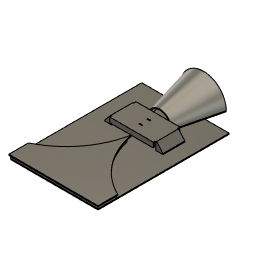
Constructed Color Sorter v1 (Autodesk Fusion 360 design; units mm, degrees)
Autodesk Fusion 360 part; units mm, degrees
sketch "Sketch1" plane through (0, 0, 0) normal (0, 1, 0) x (1, 0, 0)
  line L0 (0, 0) -> (304.8, 0)
  line L1 (304.8, 0) -> (304.8, 457.2)
  line L2 (304.8, 457.2) -> (0, 457.2)
  line L3 (0, 457.2) -> (0, 0)
  dimension "d1" = 304.8
  dimension "d2" = 457.2
  constraint horizontal L0
  constraint vertical L1
  constraint horizontal L2
  constraint vertical L3
  constraint coincident L0.start L3.end
  measures "d1" distance of L0.start L0.end
  measures "d2" distance of L0.start L2.end
extrude "Extrude1" add sketch "Sketch1" along normal blind 3.175 makes body 1
sketch "Sketch1 (2)" plane through (0, 0, 0) normal (0, 0, 1) x (1, 0, 0) in component "Ramp for Checkers v1"
  line L0 (0, 0) -> (0, 254) construction
  line L1 (0, 0) -> (152.4, 0)
  line L2 (152.4, 0) -> (152.4, 63.5)
  arc A0 (0, 254) -> (152.4, 63.5) centre (278.7714, 320.8071) ccw
  arc A1 (-152.4, 63.5) -> (0, 254) centre (-278.7714, 320.8071) ccw
  line L3 (-152.4, 0) -> (-152.4, 63.5)
  line L4 (0, 0) -> (-152.4, 0)
  dimension "d1_1" = 254
  dimension "d2_1" = 152.4
  dimension "d3_1" = 63.5
  constraint coincident L0.start L1.start
  constraint vertical L0
  constraint perpendicular L0 L1
  constraint perpendicular L1 L2
  constraint symmetric A0.start L0 A1.end
  constraint symmetric L0 L1.start L4.start
  constraint symmetric L0 L1.end L3.start
  constraint symmetric L0 L2.end A1.start
  constraint symmetric L0 A0 A1
  measures "d1_1" distance of L0.start L0.end
  measures "d2_1" distance of L0.start L1.end
  measures "d3_1" distance of L1.end L2.end
extrude "Extrude1'" add sketch "Sketch1 (2)" along normal blind 9.525 separate body makes body 2 in component "Ramp for Checkers v1"
sketch "Sketch2" plane through (0, 0, 9.525) normal (0, 0, 1) x (1, 0, 0) in component "Ramp for Checkers v1"
  line L0 (152.4, 0) -> (152.4, 63.5)
  arc A0 (0, 254) -> (152.4, 63.5) centre (278.7714, 320.8071) ccw
  arc A1 (-152.4, 63.5) -> (0, 254) centre (-278.7714, 320.8071) ccw
  line L1 (-152.4, 63.5) -> (-152.4, 0)
  line L2 (-152.4, 0) -> (152.4, 0)
  line L3 (155.575, -3.175) -> (155.575, 65.4856)
  arc A2 (0, 269.3003) -> (155.575, 65.4856) centre (278.7714, 320.8071) ccw
  arc A3 (-155.575, 65.4856) -> (0, 269.3003) centre (-278.7714, 320.8071) ccw
  line L4 (-155.575, 65.4856) -> (-155.575, -3.175)
  line L5 (-155.575, -3.175) -> (155.575, -3.175)
  dimension "d6" = -3.175
extrude "Extrude2" add sketch "Sketch2" along normal blind 3.175 contours L0 A0 A1 L1 L2 | L3 A2 A3 L4 L5 bodies 2 in component "Ramp for Checkers v1"
sketch "Sketch4" plane through (0, 0, 0) normal (0, 1, 0) x (1, 0, 0) in component "Color Sensor Mount v2"
  line L0 (0, 0) -> (152.4, 0)
  line L1 (152.4, 0) -> (152.4, 85.725)
  line L2 (152.4, 85.725) -> (0, 85.725)
  line L3 (0, 85.725) -> (0, 0)
  dimension "d16" = 152.4
  dimension "d17" = 85.725
  constraint coincident L0.start L3.end
  constraint horizontal L0
  constraint perpendicular L0 L1
  constraint perpendicular L1 L2
  constraint perpendicular L2 L3
  measures "d16" distance of L0.start L0.end
  measures "d17" distance of L0.end L1.end
extrude "Extrude4" add sketch "Sketch4" along normal blind 3.175 separate body makes body 3 in component "Color Sensor Mount v2"
sketch "Sketch5" plane through (0, 0, 0) normal (0, 0, 1) x (1, 0, 0) in component "Color Sensor Mount v2"
  line L0 (0, 0) -> (152.4, 0)
  line L1 (152.4, 0) -> (152.4, 3.175)
  line L2 (152.4, 3.175) -> (0, 3.175)
  line L3 (0, 3.175) -> (0, 0)
  line L4 (0, 3.175) -> (152.4, 3.175)
  line L5 (0, 0) -> (152.4, 0)
  line L6 (0, 0) -> (0, 3.175)
  line L7 (152.4, 0) -> (152.4, 3.175)
  line L8 (152.4, 0) -> (152.4, 17.4625)
  line L9 (0, 0) -> (0, 17.4625)
  line L10 (0, 17.4625) -> (152.4, 17.4625)
  dimension "d20" = 17.4625
  dimension "d21" = 17.4625
  constraint coincident L0.end L1.start
  constraint perpendicular L4 L8
  constraint coincident L0.start L3.end
  constraint perpendicular L4 L9
  measures "d20" distance of L0.end L8.end
  measures "d21" distance of L0.start L9.end
extrude "Extrude5" add sketch "Sketch5" along normal blind 3.175 bodies 3 in component "Color Sensor Mount v2"
sketch "Sketch6" plane through (0, 0, -85.725) normal (0, 0, -1) x (-1, 0, 0) in component "Color Sensor Mount v2"
  line L0 (-152.4, 0) -> (0, 0)
  line L1 (0, 0) -> (0, 3.175)
  line L2 (0, 3.175) -> (-152.4, 3.175)
  line L3 (-152.4, 3.175) -> (-152.4, 0)
  line L4 (-152.4, 3.175) -> (0, 3.175)
  line L5 (-152.4, 0) -> (-152.4, 3.175)
  line L6 (-152.4, 0) -> (0, 0)
  line L7 (0, 0) -> (0, 3.175)
  line L8 (0, 0) -> (0, 28.575)
  line L9 (0, 28.575) -> (-38.1, 28.575)
  line L10 (-38.1, 28.575) -> (-38.1, 12.7)
  line L11 (-38.1, 12.7) -> (-114.3, 12.7)
  line L12 (-114.3, 12.7) -> (-114.3, 28.575)
  line L13 (-114.3, 28.575) -> (-152.4, 28.575)
  line L14 (-152.4, 28.575) -> (-152.4, 0)
  dimension "d24" = 28.575
  dimension "d25" = 38.1
  dimension "d26" = 15.875
  dimension "d27" = 76.2
  dimension "d28" = 15.875
  dimension "d29" = 38.1
  constraint coincident L0.end L1.start
  constraint perpendicular L6 L8
  constraint perpendicular L8 L9
  constraint perpendicular L9 L10
  constraint perpendicular L10 L11
  constraint perpendicular L11 L12
  constraint perpendicular L12 L13
  constraint coincident L0.start L3.end
  measures "d24" distance of L0.end L8.end
  measures "d25" distance of L8.end L9.end
  measures "d26" distance of L9.end L10.end
  measures "d27" distance of L10.end L11.end
  measures "d28" distance of L11.end L12.end
  measures "d29" distance of L12.end L13.end
extrude "Extrude6" add sketch "Sketch6" along normal blind 3.175 bodies 3 in component "Color Sensor Mount v2"
sketch "Sketch7" plane through (0, 0, 0) normal (-1, 0, 0) x (0, 0, 1) in component "Color Sensor Mount v2"
  line L0 (-88.9, 0) -> (3.175, 0)
  line L1 (3.175, 0) -> (3.175, 17.4625)
  line L2 (3.175, 17.4625) -> (0, 17.4625)
  line L3 (0, 17.4625) -> (0, 3.175)
  line L4 (0, 3.175) -> (-85.725, 3.175)
  line L5 (-85.725, 3.175) -> (-85.725, 28.575)
  line L6 (-85.725, 28.575) -> (-88.9, 28.575)
  line L7 (-88.9, 28.575) -> (-88.9, 0)
  line L8 (-85.725, 3.175) -> (-85.725, 28.575)
  line L9 (-85.725, 28.575) -> (-88.9, 28.575)
  line L10 (-88.9, 0) -> (-88.9, 28.575)
  line L11 (-85.725, 3.175) -> (0, 3.175)
  line L12 (0, 3.175) -> (0, 17.4625)
  line L13 (0, 17.4625) -> (3.175, 17.4625)
  line L14 (3.175, 17.4625) -> (3.175, 0)
  line L15 (-88.9, 0) -> (3.175, 0)
  line L16 (-85.725, 3.175) -> (-80.9625, 3.175) construction
  line L17 (0, 3.175) -> (-4.7625, 3.175) construction
  line L18 (-80.9625, 0) -> (-80.9625, 28.575)
  line L19 (-4.7625, 0) -> (-4.7625, 28.575)
  line L20 (-80.9625, 28.575) -> (-4.7625, 28.575)
  dimension "d35" = 4.7625
  dimension "d36" = 4.7625
  dimension "d37" = 28.575
  dimension "d38" = 28.575
  dimension "d39" = 76.2
  constraint coincident L4.end L5.start
  constraint perpendicular L5 L16
  constraint coincident L3.end L4.start
  constraint perpendicular L12 L17
  constraint coincident L15 L18.start
  constraint perpendicular L16 L18
  constraint coincident L15 L19.start
  constraint perpendicular L11 L19
  constraint perpendicular L18 L20
  measures "d35" distance of L4.end L16.end
  measures "d36" distance of L3.end L17.end
  measures "d37" distance of L18.start L18.end
  measures "d38" distance of L19.start L19.end
  measures "d39" distance of L18.end L19.end
extrude "Extrude7" add sketch "Sketch7" along normal blind 3.175 contours L0 L4 L11 L15 L18 L19 | L4 L11 L18 L19 L20 bodies 3 in component "Color Sensor Mount v2"
sketch "Sketch8" plane through (0, 28.575, 0) normal (0, 1, 0) x (-1, 0, 0) in component "Color Sensor Mount v2"
  line L0 (0, -4.7625) -> (0, -80.9625)
  line L1 (0, -80.9625) -> (3.175, -80.9625)
  line L2 (3.175, -80.9625) -> (3.175, -4.7625)
  line L3 (3.175, -4.7625) -> (0, -4.7625)
  line L4 (0, -80.9625) -> (3.175, -80.9625)
  line L5 (0, -80.9625) -> (0, -4.7625)
  line L6 (3.175, -4.7625) -> (3.175, -80.9625)
  line L7 (0, -4.7625) -> (3.175, -4.7625)
  line L8 (0, -4.7625) -> (25.4, -4.7625)
  line L9 (0, -80.9625) -> (25.4, -80.9625)
  line L10 (25.4, -80.9625) -> (25.4, -4.7625)
  dimension "d42" = 25.4
  dimension "d43" = 25.4
  dimension "d44" = 76.2
  constraint coincident L0.start L3.end
  constraint perpendicular L5 L8
  constraint coincident L0.end L1.start
  constraint perpendicular L5 L9
  constraint perpendicular L8 L10
  measures "d42" distance of L0.start L8.end
  measures "d43" distance of L0.end L9.end
  measures "d44" distance of L9.end L8.end
extrude "Extrude9" add sketch "Sketch8" against normal blind 3.175 contours L2 L6 L8 L9 L10 bodies 3 in component "Color Sensor Mount v2"
ref_plane "WorkPlane1" through (76.2, 14.2875, -42.8625) normal (1, 0, 0) x (0, 0, -1) in component "Color Sensor Mount v2"
mirror "Mirror1" about plane through (76.2, 14.2875, -42.8625) normal (1, 0, 0) of "Extrude7" in component "Color Sensor Mount v2"
mirror "Mirror3" about plane through (76.2, 14.2875, -42.8625) normal (1, 0, 0) of "Extrude9" in component "Color Sensor Mount v2"
sketch "Sketch9" plane through (0, 0, -80.9625) normal (0, 0, -1) x (-1, 0, 0) in component "Color Sensor Mount v2"
  line L0 (-152.4, 0) -> (-152.4, 3.175)
  line L1 (-152.4, 3.175) -> (-152.4, 28.575)
  line L2 (-152.4, 28.575) -> (-177.8, 28.575)
  line L3 (-177.8, 28.575) -> (-177.8, 25.4)
  line L4 (-177.8, 25.4) -> (-155.575, 25.4)
  line L5 (-155.575, 25.4) -> (-155.575, 0)
  line L6 (-155.575, 0) -> (-152.4, 0)
  line L7 (-177.8, 25.4) -> (-155.575, 0)
  constraint coincident L3.end L4.start
  constraint coincident L5.end L6.start
extrude "Extrude10" add sketch "Sketch9" against normal up to surface (76.2 mm away) contours L4 L5 L7 bodies 3 in component "Color Sensor Mount v2"
mirror "Mirror4" about plane through (76.2, 14.2875, -42.8625) normal (1, 0, 0) of "Extrude10" in component "Color Sensor Mount v2"
sketch "Sketch10" plane through (0, 3.175, 0) normal (0, 1, 0) x (-1, 0, 0) in component "Color Sensor Mount v2"
  line L0 (0, -85.725) -> (0, -80.9625)
  line L1 (0, -80.9625) -> (0, -4.7625)
  line L2 (0, -4.7625) -> (0, 0)
  line L3 (0, 0) -> (-152.4, 0)
  line L4 (-152.4, 0) -> (-152.4, -4.7625)
  line L5 (-152.4, -4.7625) -> (-152.4, -80.9625)
  line L6 (-152.4, -80.9625) -> (-152.4, -85.725)
  line L7 (-152.4, -85.725) -> (0, -85.725)
  line L8 (0, -80.9625) -> (0, -4.7625)
  line L9 (-152.4, -85.725) -> (0, -85.725)
  line L10 (0, -85.725) -> (0, -80.9625)
  line L11 (0, -4.7625) -> (0, 0)
  line L12 (0, 0) -> (-152.4, 0)
  line L13 (-152.4, -4.7625) -> (-152.4, -80.9625)
  line L14 (-152.4, -80.9625) -> (-152.4, -85.725)
  line L15 (-152.4, 0) -> (-152.4, -4.7625)
  line L16 (0, -85.725) -> (-152.4, 0) construction
  line L17 (-152.4, -85.725) -> (0, 0) construction
  line L18 (-76.2, -42.8625) -> (-88.2955, -42.8625) construction
  line L19 (-76.2, -42.8625) -> (-64.1096, -42.8625) construction
  line L20 (-64.1096, -42.8625) -> (-64.1096, -58.3692) construction
  line L21 (-64.1096, -42.8625) -> (-64.1096, -27.3558) construction
  line L22 (-64.1096, -58.3692) -> (-88.2904, -58.3692) construction
  line L23 (-64.1096, -27.3558) -> (-88.2904, -27.3558) construction
  line L24 (-88.2904, -58.3692) -> (-88.2904, -27.3558) construction
  line L25 (-64.1096, -58.3692) -> (-71.12, -58.3692) construction
  line L26 (-88.2904, -58.3692) -> (-81.28, -58.3692) construction
  line L27 (-64.1096, -27.3558) -> (-71.12, -27.3558) construction
  line L28 (-71.12, -58.3692) -> (-71.12, -55.8292)
  line L29 (-71.12, -55.8292) -> (-81.28, -55.8292)
  line L30 (-81.28, -55.8292) -> (-81.28, -58.3692)
  line L31 (-71.12, -58.3692) -> (-81.28, -58.3692)
  line L32 (-71.12, -27.3558) -> (-71.12, -29.8958)
  line L33 (-71.12, -29.8958) -> (-81.28, -29.8958)
  line L34 (-81.28, -29.8958) -> (-81.28, -27.3558)
  line L35 (-64.1096, -27.3558) -> (-88.2904, -27.3558) construction
  line L36 (-71.12, -27.3558) -> (-81.28, -27.3558)
  point P0 (-152.4, -85.725)
  dimension "d61" = 15.5067
  dimension "d62" = 15.5067
  dimension "d63" = 24.1808
  dimension "d64" = 7.0104
  dimension "d65" = 7.0104
  dimension "d66" = 2.54
  constraint coincident L0.start L7.end
  constraint coincident L3.end L4.start
  constraint coincident P0 L6.end
  constraint coincident L2.end L3.start
  constraint midpoint L17 L18.start
  constraint perpendicular L8 L18
  constraint parallel L18 L19
  constraint perpendicular L19 L20
  constraint perpendicular L19 L21
  constraint perpendicular L20 L22
  constraint perpendicular L21 L23
  constraint perpendicular L23 L24
  constraint coincident L22 L25.end
  constraint perpendicular L24 L26
  constraint symmetric L19 L20.end L21.end
  constraint symmetric L19 L25.end L27.end
  constraint perpendicular L22 L28
  constraint perpendicular L28 L29
  constraint perpendicular L26 L30
  constraint symmetric L19 L22.end L23.end
  constraint symmetric L19 L26.end L34.end
  constraint symmetric L19 L28.end L32.end
  constraint symmetric L19 L29.end L33.end
  measures "d61" distance of L19.end L20.end
  measures "d62" distance of L19.end L21.end
  measures "d63" distance of L20.end L22.end
  measures "d64" distance of L20.end L25.end
  measures "d65" distance of L22.end L26.end
  measures "d66" distance of L25.end L28.end
extrude "Extrude11" cut sketch "Sketch10" against normal blind 14.7066 contours L28 L29 L30 L31 | L32 L33 L34 L36 bodies 3 in component "Color Sensor Mount v2"
move_body "Move1" bodies 3 to x (1, 0, 0) y (0, 0, 1) z (0, -1, 0) at (0, 20.6375, -14.2875) in component "Color Sensor Mount v2"
sketch "Sketch11" plane through (0, 109.5375, 0) normal (0, 1, 0) x (-1, 0, 0) in component "Color Sensor Mount v2"
  line L0 (-152.4, 14.2875) -> (-152.4, -14.2875)
  line L1 (-152.4, -14.2875) -> (0, -14.2875)
  line L2 (0, -14.2875) -> (0, 14.2875)
  line L3 (0, 14.2875) -> (-38.1, 14.2875)
  line L4 (-38.1, 14.2875) -> (-38.1, -1.5875)
  line L5 (-38.1, -1.5875) -> (-114.3, -1.5875)
  line L6 (-114.3, -1.5875) -> (-114.3, 14.2875)
  line L7 (-114.3, 14.2875) -> (-152.4, 14.2875)
  line L8 (-114.3, 14.2875) -> (-38.1, 14.2875) construction
  constraint coincident L6.end L7.start
  constraint coincident L3.end L4.start
sketch "Sketch12" plane through (0, 109.5375, 0) normal (0, 1, 0) x (-1, 0, 0) in component "Color Sensor Mount v2"
  line L0 (-152.4, 14.2875) -> (-152.4, -14.2875)
  line L1 (-152.4, -14.2875) -> (0, -14.2875)
  line L2 (0, -14.2875) -> (0, 14.2875)
  line L3 (0, 14.2875) -> (-38.1, 14.2875)
  line L4 (-38.1, 14.2875) -> (-38.1, -1.5875)
  line L5 (-38.1, -1.5875) -> (-114.3, -1.5875)
  line L6 (-114.3, -1.5875) -> (-114.3, 14.2875)
  line L7 (-114.3, 14.2875) -> (-152.4, 14.2875)
sketch "Sketch2 (2)" plane through (0, -0.4135, 0) normal (0, 1, 0) x (-1, 0, 0)
  line L0 (-451.4462, -73.2838) -> (-603.8462, -73.2838)
  line L1 (-603.8462, -73.2838) -> (-603.8462, -90.7463)
  line L2 (-603.8462, -90.7463) -> (-451.4462, -90.7463)
  line L3 (-451.4462, -90.7463) -> (-451.4462, -73.2838)
  line L4 (-451.4462, -73.2838) -> (-603.8462, -73.2838)
  line L5 (-603.8462, -73.2838) -> (-603.8462, -90.7463)
  line L6 (-603.8462, -90.7463) -> (-451.4462, -90.7463)
  line L7 (-451.4462, -90.7463) -> (-451.4462, -73.2838)
  line L8 (-451.4462, -73.2838) -> (-451.4462, -101.8588)
  line L9 (-451.4462, -101.8588) -> (-603.8462, -101.8588)
  line L10 (-603.8462, -90.7463) -> (-603.8462, -101.8588)
  dimension "d5" = 28.575
  constraint coincident L0.start L3.end
  constraint perpendicular L4 L8
  constraint perpendicular L5 L9
  constraint coincident L1.end L2.start
  constraint perpendicular L9 L10
  measures "d5" distance of L0.start L8.end
sketch "Sketch3" plane through (0, 0, 0) normal (0, 0, 1) x (1, 0, 0)
sketch "Sketch1 (3)" plane through (0, 0, 0) normal (0, 0, 1) x (1, 0, 0) in component "Checker Feeeder v2"
  line L0 (0, 0) -> (38.1, 0) construction
  line L1 (0, 0) -> (0, 152.4) construction
  line L2 (0, 152.4) -> (76.2, 152.4) construction
  line L3 (76.2, 152.4) -> (38.1, 0)
  line L4 (79.4727, 152.4) -> (41.3727, 0)
  line L5 (38.1, 0) -> (41.3727, 0)
  line L6 (76.2, 152.4) -> (79.4727, 152.4)
  dimension "d1_2" = 38.1
  dimension "d2_2" = 152.4
  dimension "d3_2" = 76.2
  constraint coincident L0.start L1.start
  constraint horizontal L0
  constraint perpendicular L0 L1
  constraint perpendicular L1 L2
  constraint parallel L0 L5
  constraint parallel L3 L4
  constraint parallel L2 L6
  measures "d1_2" distance of L0.start L0.end
  measures "d2_2" distance of L0.start L1.end
  measures "d3_2" distance of L1.end L2.end
revolve "Revolve1" add sketch "Sketch1 (3)" angle 180 about axis through (0, 0, 0) along (0, -1, 0) separate body makes body 4 in component "Checker Feeeder v2"
sketch "Sketch2 (3)" plane through (0, 0, 0) normal (0, 0, -1) x (-1, 0, 0) in component "Checker Feeeder v2"
  line L0 (-41.3727, 0) -> (-38.1, 0)
  line L1 (-38.1, 0) -> (-76.2, 152.4)
  line L2 (-76.2, 152.4) -> (-79.4727, 152.4)
  line L3 (-79.4727, 152.4) -> (-41.3727, 0)
  line L4 (38.1, 0) -> (41.3727, 0)
  line L5 (41.3727, 0) -> (79.4727, 152.4)
  line L6 (79.4727, 152.4) -> (76.2, 152.4)
  line L7 (76.2, 152.4) -> (38.1, 0)
  line L8 (-76.2, 152.4) -> (76.2, 152.4)
  line L9 (-38.1, 0) -> (38.1, 0)
  line L10 (-79.4727, 152.4) -> (79.4727, 152.4)
  line L11 (-41.3727, 0) -> (41.3727, 0)
  line L12 (79.4727, 152.4) -> (41.3727, 0)
  line L13 (-79.4727, 152.4) -> (-41.3727, 0)
  constraint coincident L2.end L3.start
  constraint coincident L5.end L6.start
  constraint coincident L0.start L3.end
  constraint coincident L4.end L5.start
extrude "Extrude2'" add sketch "Sketch2 (3)" along normal blind 3.175 bodies 4 in component "Checker Feeeder v2"
move_body "Move1'" bodies 4 to x (1, 0, 0) y (0, 0, -1) z (0, 1, 0) at (0, 3.175, -3.175) in component "Checker Feeeder v2"
move_body "Move2" bodies 4 to x (0, 0, 1) y (0, 1, 0) z (-1, 0, 0) at (0, 0, 0) in component "Checker Feeeder v2"
component "Ramp for Checkers v1" placed x (1, 0, 0) y (0, 0, -1) z (0, 1, 0) at (152.4, 3.175, 0)
component "Color Sensor Mount v2" placed x (-1, 0, 0) y (0, 0, -1) z (0, -1, 0) at (228.6, 17.4625, -251.8378)
component "Checker Feeeder v2" placed x (0, 0, -1) y (0, 1, 0) z (1, 0, 0) at (155.575, 3.175, -361.3753)
equation "d1 = 12\""
equation "d2 = 18\""
equation "d1_1 = 10\""
equation "d2_1 = 6\""
equation "d16 = 6\""
equation "d27 = 3\""
equation "d39 = 3\""
equation "d42 = 1\""
equation "d43 = 1\""
equation "d44 = 3\""
equation "d63 = ( 0.476 in + 0.476 in )"
equation "d1_2 = ( 3 / 2 ) * 1 in"
